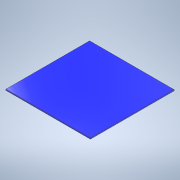
# Autodesk Inventor part: ETL Sensor
Saved by Autodesk Inventor 2022 (Build 260153000, 153)
## iProperties
Created: 2022-02-01
Part Number: ETL Sensor
Material: Silicon Nitride
Document SubType Name: Modeling
Designer: Caleb
Density: 3.18 g/cm^3
Appearance: Chrome - Polished Black
Author: Caleb
Autodesk Inventor part; units mm, degrees
ref_plane "YZ Plane" through (0, 0, 0) normal (1, 0, 0) x (0, 1, 0)
ref_plane "XZ Plane" through (0, 0, 0) normal (0, 1, 0) x (-1, 0, 0)
ref_plane "XY Plane" through (0, 0, 0) normal (0, 0, 1) x (1, 0, 0)
sketch "Sketch1" plane through (0, 0, 0) normal (0, 1, 0) x (-1, 0, 0)
  line L0 (-10.8, 10.7) -> (10.8, 10.7)
  line L1 (10.8, 10.7) -> (10.8, -10.7)
  line L2 (10.8, -10.7) -> (-10.8, -10.7)
  line L3 (-10.8, -10.7) -> (-10.8, 10.7)
  line L4 (-10.8, 10.7) -> (10.8, -10.7) construction
  line L5 (10.8, 10.7) -> (-10.8, -10.7) construction
  point P0 (0, 0)
  dimension "d0" = 21.4
  dimension "d1" = 21.6
  constraints: 12 end point, 2 midpoint, 2 parallel, 1 horizontal, 1 perpendicular
  measures "d0" distance of L0.end L1.end
  measures "d1" distance of L1.end L2.end
extrude "Extrusion1" add sketch "Sketch1" along normal blind 0.3
body "Solid1"
